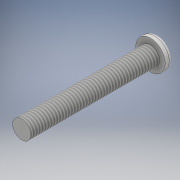
# Autodesk Inventor part: M5x35mm-crosshead
Saved by Autodesk Inventor 2018 (Build 220112000, 112)
## iProperties
Created: 2017-10-15
Part Number: M5x35mm-crosshead
Material: Generic
Document SubType Name: Modeling
Designer: Jurjen
Density: 1 g/cm^3
Appearance: Default
Author: Jurjen
Autodesk Inventor part; units mm, degrees
ref_plane "YZ Plane" through (0, 0, 0) normal (1, 0, 0) x (0, 1, 0)
ref_plane "XZ Plane" through (0, 0, 0) normal (0, 1, 0) x (-1, 0, 0)
ref_plane "XY Plane" through (0, 0, 0) normal (0, 0, 1) x (1, 0, 0)
sketch "Sketch1" plane through (0, 0, 0) normal (0, 0, 1) x (1, 0, 0)
  line L0 (2.5, 16.45) -> (2.5, -18.55)
  line L1 (2.5, -18.55) -> (0, -18.55)
  line L2 (0, -18.55) -> (0, 18.55)
  line L3 (0, 18.55) -> (4, 18.55)
  line L4 (4, 18.55) -> (4, 16.45)
  line L5 (4, 16.45) -> (2.5, 16.45)
  point P0 (0, 0)
  point P1 (0, 0)
  dimension "d0" = 2.5
  dimension "d1" = 35
  dimension "d2" = 2.1
  dimension "d3" = 4
  constraints: 12 end point, 5 perpendicular, 1 coincident, 1 midpoint, 1 vertical, 1 vertical alignment
  measures "d0" distance between parallel lines of L2 L0
  measures "d1" distance of L0.start L0.end
  measures "d2" distance between parallel lines of L5 L3
  measures "d3" distance of L2.end L3.end
revolve "Revolution1" add sketch "Sketch1" angle 360 about axis through (0, -18.55, 0) along (0, 1, 0)
fillet "Fillet1" radius 1 1 edges at (-4, 18.55, 0)
sketch "Sketch2" plane through (0, 18.55, 0) normal (0, 1, 0) x (1, 0, 0)
  line L0 (-2.7, 0) -> (-2.7, -0.75)
  line L1 (-2.7, -0.75) -> (-0.75, -0.75)
  line L2 (-0.75, -0.75) -> (-0.75, -2.7)
  line L3 (-0.75, -2.7) -> (0, -2.7)
  line L4 (2.7, -0.75) -> (2.7, 0)
  line L5 (0.75, -2.7) -> (0.75, -0.75)
  line L6 (0, -2.7) -> (0.75, -2.7)
  line L7 (0.75, -0.75) -> (2.7, -0.75)
  line L8 (0.75, 2.7) -> (0, 2.7)
  line L9 (2.7, 0.75) -> (0.75, 0.75)
  line L10 (2.7, 0) -> (2.7, 0.75)
  line L11 (0.75, 0.75) -> (0.75, 2.7)
  line L12 (-2.7, 0.75) -> (-2.7, 0)
  line L13 (-0.75, 2.7) -> (-0.75, 0.75)
  line L14 (0, 2.7) -> (-0.75, 2.7)
  line L15 (-0.75, 0.75) -> (-2.7, 0.75)
  line L16 (-0.75, -2.7) -> (0.75, -2.7)
  line L17 (2.7, -0.75) -> (2.7, 0.75)
  line L18 (-0.75, 2.7) -> (0.75, 2.7)
  line L19 (-2.7, -0.75) -> (-2.7, 0.75)
  point P0 (0, 0)
  dimension "d6" = 0.75
  dimension "d7" = 0.75
  dimension "d8" = 2.7
  dimension "d9" = 2.7
  dimension "d12" = 360
  constraints: 40 end point, 4 perpendicular, 1 horizontal alignment, 1 vertical, 1 vertical alignment, 37 other
  measures "d6" distance from line of point (0, 0) L1
  measures "d7" distance from line of point (0, 0) L2
  measures "d8" distance from line of point (0, 0) L3
  measures "d9" distance from line of point (0, 0) L0
extrude "Extrusion1" cut sketch "Sketch2" against normal blind 1
thread "Thread1" size "M5x0.8" class "6g" standard "ANSI Metric M Profile" full length
equation "\"d9\" = d8"
body "Solid1"
